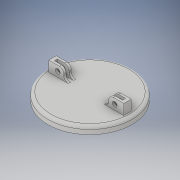
# Autodesk Inventor part: Main PCB Base
Saved by Autodesk Inventor 2018.3 (Build 223284000, 284)
## iProperties
Company: UNH Makerspace
Created: 2019-07-26
Part Number: Main PCB Base
Material: Generic
Document SubType Name: Modeling
Designer: Electro707
Density: 1 g/cm^3
Appearance: Default
Engineer: Jamal Bouajjaj
Description: The base for the main PCB
Author: Electro707
Title: Dual Construction Tree - Base
Revision Number: N/A
Autodesk Inventor part; units mm, degrees
ref_plane "YZ Plane" through (0, 0, 0) normal (1, 0, 0) x (0, 1, 0)
ref_plane "XZ Plane" through (0, 0, 0) normal (0, 1, 0) x (-1, 0, 0)
ref_plane "XY Plane" through (0, 0, 0) normal (0, 0, 1) x (1, 0, 0)
sketch "Sketch1" plane through (0, 0, 0) normal (0, 0, 1) x (1, 0, 0)
  line L0 (25, 7) -> (-25, 7)
  line L1 (-25, 7) -> (-25, 0)
  line L2 (-25, 0) -> (25, 0)
  line L3 (25, 0) -> (25, 7)
  circle A0 centre (-19, 3.5) radius 1.6
  circle A1 centre (19, 3.5) radius 1.6
  line L4 (19, 3.5) -> (-19, 3.5) construction
  line L5 (19, 3.5) -> (25, 7) construction
  line L6 (19, 3.5) -> (25, 0) construction
  line L7 (-19, 3.5) -> (-25, 7) construction
  line L8 (-19, 3.5) -> (-25, 0) construction
  line L9 (0, 0) -> (-19, 3.5) construction
  line L10 (0, 0) -> (19, 3.5) construction
  dimension "d0" = 3.2
  dimension "d1" = 38
  dimension "d2" = 7
  dimension "d3" = 50
  constraints: 22 end point, 4 equal length, 2 centre point, 2 horizontal, 2 parallel, 1 equal radius, 1 midpoint, 1 perpendicular
  measures "d0" diameter of A1
  measures "d1" distance of L4.start L4.end
  measures "d2" distance of L0.end L1.end
  measures "d3" distance of L0.start L0.end
extrude "Extrusion1" add sketch "Sketch1" along normal blind 5
sketch "Sketch2" plane through (-25, 7, 0) normal (0, 1, 0) x (1, 0, 0)
  line L0 (2.25, -3.5) -> (10, -3.5)
  line L1 (47.75, -3.5) -> (47.75, -1.5)
  line L2 (47.75, -1.5) -> (40, -1.5)
  line L3 (2.25, -1.5) -> (2.25, -3.5)
  line L4 (50, -5) -> (0, -5) construction
  line L5 (0, -5) -> (2.25, -3.5) construction
  line L6 (50, 0) -> (0, 0) construction
  line L7 (2.25, -1.5) -> (0, 0) construction
  line L8 (50, 0) -> (50, -5) construction
  line L9 (47.75, -3.5) -> (50, -5) construction
  line L10 (40, -3.5) -> (40, -5)
  line L11 (40, -5) -> (10, -5)
  line L12 (10, -5) -> (10, -3.5)
  line L13 (10, -1.5) -> (10, 0)
  line L14 (10, 0) -> (40, 0)
  line L15 (40, 0) -> (40, -1.5)
  line L16 (40, -3.5) -> (47.75, -3.5)
  line L17 (40, -1.5) -> (10, -1.5) construction
  line L18 (10, -3.5) -> (40, -3.5) construction
  line L19 (10, -1.5) -> (2.25, -1.5)
  line L20 (47.75, -3.5) -> (40, -5) construction
  line L21 (40, 0) -> (47.75, -1.5) construction
  line L22 (10, -5) -> (2.25, -3.5) construction
  line L23 (2.25, -1.5) -> (10, 0) construction
  point P0 (25, 0)
  dimension "d6" = 45.5
  dimension "d7" = 2
  dimension "d13" = 30
  constraints: 42 end point, 10 parallel, 9 perpendicular, 6 point on line, 5 equal length, 3 horizontal, 2 collinear
  measures "d6" distance of L1.end L3.start
  measures "d7" distance of L3.start L0.start
  measures "d13" distance of L10.end L11.end
extrude "Extrusion2" cut sketch "Sketch2" against normal up to next
sketch "Sketch3" plane through (-25, 0, 0) normal (0, -1, 0) x (1, 0, 0)
  circle A0 centre (25, 2.5) radius 28
  line L0 (0, 5) -> (50, 5) construction
  line L1 (0, 5) -> (25, 2.5) construction
  line L2 (0, 0) -> (50, 0) construction
  line L3 (25, 2.5) -> (0, 0) construction
  line L4 (25, 2.5) -> (50, 5) construction
  point P0 (25, 0)
  dimension "d10" = 56
  constraints: 6 end point, 2 equal length, 1 centre point
  measures "d10" diameter of A0
extrude "Extrusion3" add sketch "Sketch3" along normal blind 5
fillet "Fillet1" radius 3 8 edges at (15, 7, 0.75) (15, 7, 4.25) (15, 0, 4.25) (15, 0, 0.75) (-15, 0, 0.75) (-15, 7, 0.75) (-15, 7, 4.25) (-15, 0, 4.25)
fillet "Fillet2" radius 2 1 edges at (-28, 0, 2.5)
body "Solid1"
